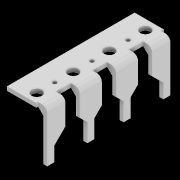
# Autodesk Inventor part: suporte 555
Saved by Autodesk Inventor 2020 (Build 240168000, 168)
## iProperties
Created: 2020-02-11
Part Number: suporte 555
Material: Generic
Document SubType Name: Modeling
Designer: PEDRO
Density: 1 g/cm^3
Appearance: Default
Author: PEDRO
Autodesk Inventor part; units mm, degrees
ref_plane "YZ Plane" through (0, 0, 0) normal (1, 0, 0) x (0, 1, 0)
sketch "Sketch1" plane through (0, 0, 0) normal (0, 1, 0) x (-1, 0, 0)
  line L0 (0, 0) -> (22.85, 0)
  line L1 (22.85, 0) -> (22.85, -100)
  line L2 (22.85, -100) -> (0, -100)
  line L3 (0, -100) -> (0, 0)
  circle A0 centre (6.72, -92.29) radius 4
  circle A1 centre (6.72, -64.05) radius 4
  circle A2 centre (6.72, -35.65) radius 4
  circle A3 centre (6.72, -7.1) radius 4
  circle A4 centre (6.72, -21.17) radius 1.5
  circle A5 centre (6.72, -50.38) radius 1.5
  circle A6 centre (6.72, -78.72) radius 1.5
  line L4 (6.72, -7.1) -> (-10.3799, -7.1) construction
  line L5 (6.72, -35.65) -> (-7.55, -35.65) construction
  line L6 (6.72, -64.05) -> (-7.55, -64.05) construction
  line L7 (6.72, -92.29) -> (-7.55, -92.29) construction
  line L8 (0, -27.127) -> (-7.15, -27.127)
  line L9 (0, -44.173) -> (-7.15, -44.173)
  line L10 (0, -55.527) -> (-7.15, -55.527)
  line L11 (0, -72.573) -> (-7.15, -72.573)
  line L12 (0, -83.767) -> (-7.15, -83.767)
  line L13 (0, -97.95) -> (-7.15, -97.95)
  line L14 (0, -1.44) -> (-7.15, -1.44)
  line L15 (0, -15.623) -> (-7.15, -15.623)
  line L16 (-7.15, -1.44) -> (-7.15, -15.623)
  line L17 (-7.15, -27.127) -> (-7.15, -44.173)
  line L18 (-7.15, -55.527) -> (-7.15, -72.573)
  line L19 (-7.15, -83.767) -> (-7.15, -97.95)
  line L20 (-7.15, 0) -> (-7.15, -100) construction
  dimension "d0" = 22.85
  dimension "d1" = 100
  dimension "d2" = 8
  dimension "d3" = 8
  dimension "d4" = 8
  dimension "d5" = 8
  dimension "d7" = 0
  dimension "d8" = 0
  dimension "d9" = 0
  dimension "d14" = 3
  dimension "d15" = 3
  dimension "d16" = 3
  dimension "d17" = 6.72
  dimension "d18" = 6.72
  dimension "d19" = 0
  dimension "d20" = 0
  dimension "d28" = 8.523
  dimension "d29" = 8.523
  dimension "d30" = 8.523
  dimension "d31" = 8.523
  dimension "d32" = 8.523
  dimension "d33" = 5.66
  dimension "d34" = 5.66
  dimension "d35" = 8.523
  dimension "d36" = 100
  dimension "d42" = 7.15
  dimension "d80" = 7.71
  dimension "d81" = 35.95
  dimension "d82" = 64.35
  dimension "d83" = 92.9
  dimension "d84" = 21.28
  dimension "d85" = 49.62
  dimension "d86" = 78.83
  constraints: 40 end point, 9 parallel, 7 centre point, 5 perpendicular, 4 point on line, 3 vertical, 2 collinear, 2 horizontal, 11 other
  measures "d0" distance of L1.end L2.end
  measures "d1" distance of L0.end L1.end
  measures "d2" diameter of A0
  measures "d3" diameter of A1
  measures "d4" diameter of A2
  measures "d5" diameter of A3
  measures "d7" horizontal distance of L4.start L5.start
  measures "d8" horizontal distance of L4.start L6.start
  measures "d9" horizontal distance of L4.start L7.start
  measures "d14" diameter of A4
  measures "d15" diameter of A5
  measures "d16" diameter of A6
  measures "d19" horizontal distance of A4.centre A5.centre
  measures "d20" horizontal distance of A5.centre A6.centre
  measures "d28" distance between parallel lines of L5 L8
  measures "d29" distance between parallel lines of L5 L9
  measures "d30" distance between parallel lines of L6 L10
  measures "d31" distance between parallel lines of L6 L11
  measures "d32" distance between parallel lines of L7 L12
  measures "d33" distance between parallel lines of L7 L13
  measures "d34" distance between parallel lines of L4 L14
  measures "d35" distance between parallel lines of L4 L15
  measures "d36" distance of L20.start L20.end
  measures "d42" distance of the line from the sketch origin of L20
  measures "d80" distance from line of L2 L7.start
  measures "d81" distance from line of L2 L6.start
  measures "d82" distance from line of L2 L5.start
  measures "d83" distance from line of L2 L4.start
  measures "d84" distance from line of L2 A6.centre
  measures "d85" distance from line of L2 A5.centre
  measures "d86" distance from line of L2 A4.centre
extrude "Extrusion1" add sketch "Sketch1" against normal blind 3
ref_plane "Work Plane2" through (7.15, 0, -15.623) normal (1, 0, 0) x (0, 0, -1)
ref_plane "Work Plane3" through (7.15, 0, -1.44) normal (1, 0, 0) x (0, 0, -1)
sketch "Sketch3" plane through (7.15, 0, -1.44) normal (1, 0, 0) x (0, 0, -1)
  line L0 (0, 0) -> (14.183, 0) projected
  line L1 (14.183, -3) -> (0, -3) projected
  line L2 (14.183, 0) -> (14.183, -3) projected
  line L3 (0, 0) -> (0, -3) projected
  line L4 (25.687, 0) -> (42.733, 0) projected
  line L5 (25.687, 0) -> (25.687, -3) projected
  line L6 (42.733, -3) -> (25.687, -3) projected
  line L7 (42.733, 0) -> (42.733, -3) projected
  line L8 (54.087, 0) -> (71.133, 0) projected
  line L9 (54.087, 0) -> (54.087, -3) projected
  line L10 (71.133, -3) -> (54.087, -3) projected
  line L11 (71.133, 0) -> (71.133, -3) projected
  line L12 (82.327, 0) -> (96.51, 0) projected
  line L13 (82.327, 0) -> (82.327, -3) projected
  line L14 (96.51, -3) -> (82.327, -3) projected
  line L15 (96.51, 0) -> (96.51, -3) projected
  line L16 (0, 0) -> (0, -40)
  line L17 (0, -40) -> (5.4, -40)
  line L18 (14.183, 0) -> (14.183, -20)
  line L19 (5.4, -40) -> (5.4, -28.783)
  line L20 (14.183, -20) -> (5.4, -28.783)
  line L21 (71.133, 0) -> (71.133, -20)
  line L22 (54.087, 0) -> (54.087, -20)
  line L23 (71.133, -20) -> (65.31, -25.823)
  line L24 (65.31, -25.823) -> (65.31, -40)
  line L25 (65.31, -40) -> (59.91, -40)
  line L26 (59.91, -40) -> (59.91, -25.823)
  line L27 (59.91, -25.823) -> (54.087, -20)
  line L28 (62.61, -40) -> (62.61, 0) construction
  line L29 (54.087, 0) -> (71.133, 0) projected
  line L30 (42.733, 0) -> (42.733, -20)
  line L31 (25.687, 0) -> (25.687, -20)
  line L32 (42.733, -20) -> (36.91, -25.823)
  line L33 (36.91, -25.823) -> (36.91, -40)
  line L34 (36.91, -40) -> (31.51, -40)
  line L35 (31.51, -40) -> (31.51, -25.823)
  line L36 (31.51, -25.823) -> (25.687, -20)
  line L37 (34.21, -40) -> (34.21, 0) construction
  line L38 (98.56, 0) -> (-1.44, 0) projected
  line L39 (96.51, 0) -> (96.51, -40)
  line L40 (96.51, -40) -> (91.11, -40)
  line L41 (91.11, -40) -> (91.11, -28.783)
  line L42 (91.11, -28.783) -> (82.327, -20)
  line L43 (82.327, 0) -> (82.327, -3) projected
  line L44 (82.327, -20) -> (82.327, 0)
  point P0 (25.687, -3)
  point P1 (14.183, -3)
  point P2 (96.51, -3)
  dimension "d46" = 40
  dimension "d47" = 5.4
  dimension "d48" = 20
  dimension "d51" = 135
  dimension "d61" = 20
  dimension "d62" = 135
  dimension "d63" = 135
  dimension "d64" = 5.4
  dimension "d66" = 20
  dimension "d67" = 20
  dimension "d68" = 135
  dimension "d69" = 135
  dimension "d70" = 5.4
  dimension "d71" = 20
  dimension "d89" = 5.4
  dimension "d90" = 40
  dimension "d91" = 135
  dimension "d92" = 20
  constraints: 52 end point, 10 vertical, 8 perpendicular, 5 collinear, 4 midpoint, 1 horizontal, 1 other
  measures "d46" distance of L0.start L16.end
  measures "d47" distance of L16.end L17.end
  measures "d48" distance of L0.end L18.end
  measures "d51" angle of L18 L20
  measures "d61" distance of L8.end L21.end
  measures "d62" angle of L22 L27
  measures "d63" angle of L21 L23
  measures "d64" distance of L24.end L25.end
  measures "d66" distance of L8.start L22.end
  measures "d67" distance of L4.end L30.end
  measures "d68" angle of L31 L36
  measures "d69" angle of L30 L32
  measures "d70" distance of L34.start L34.end
  measures "d71" distance of L4.start L36.end
  measures "d89" distance of L39.end L40.end
  measures "d90" distance of L12.end L39.end
  measures "d91" angle of L44 L42
  measures "d92" distance of L42.end L12.start
extrude "Extrusion3" add sketch "Sketch3" against normal blind 3
chamfer "Chamfer2" distance 4 angle 45 4 edges at (4.15, -3, -90.8585) (4.15, -3, -64.05) (4.15, -3, -35.65) (4.15, -3, -8.5315)
fillet "Fillet2" radius 4 4 edges at (7.15, 0, -8.5315) (7.15, 0, -35.65) (7.15, 0, -64.05) (7.15, 0, -90.8585)
equation "\"d18\" = d17"
body "Solid1"
